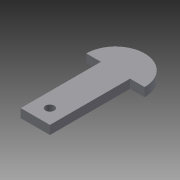
# Autodesk Inventor part: fixing
Saved by Autodesk Inventor 2015 SP2 (Build 190223200, 223)
## iProperties
Created: 2016-03-17
Part Number: fixing
Material: Generic
Document SubType Name: Modeling
Designer: mca20
Density: 1 g/cm^3
Appearance: Default
Author: mca20
Autodesk Inventor part; units mm, degrees
ref_plane "YZ Plane" through (0, 0, 0) normal (1, 0, 0) x (0, 1, 0)
ref_plane "XZ Plane" through (0, 0, 0) normal (0, 1, 0) x (-1, 0, 0)
ref_plane "XY Plane" through (0, 0, 0) normal (0, 0, 1) x (1, 0, 0)
sketch "Sketch1" plane through (0, 0, 0) normal (0, 1, 0) x (-1, 0, 0)
  line L0 (0, 0) -> (10, 0)
  line L1 (10, 0) -> (10, -27.5)
  line L2 (10, -27.5) -> (0, -27.5)
  line L3 (0, -27.5) -> (0, 0)
  line L4 (10, -27.5) -> (15, -27.5)
  line L5 (0, -27.5) -> (-5, -27.5)
  arc A0 (-5, -27.5) -> (15, -27.5) centre (5, -27.5143) ccw
  dimension "d0" = 10
  dimension "d1" = 27.5
  dimension "d2" = 5
  dimension "d3" = 5
  constraints: 12 end point, 2 horizontal, 2 parallel, 2 point on circle, 1 centre point, 1 perpendicular, 1 point on line
  measures "d0" distance of L1.end L2.end
  measures "d1" distance of L0.end L1.end
  measures "d2" distance of L1.end L4.end
  measures "d3" distance of L2.end L5.end
extrude "Extrusion1" add sketch "Sketch1" along normal blind 3
sketch "Sketch2" plane through (0, 3, 0) normal (0, 1, 0) x (1, 0, 0)
  circle A0 centre (-5, 5) radius 1.5
  line L0 (-10, 0) -> (0, 0) projected
  line L1 (-10, 27.5) -> (-10, 0) projected
  dimension "d6" = 3
  dimension "d7" = 5
  dimension "d8" = 5
  constraints: 1 centre point
  measures "d6" diameter of A0
  measures "d7" distance from line of L0 A0.centre
  measures "d8" distance from line of L1 A0.centre
hole "Hole1" at (-5, 3, -5) direction (0, -1, 0) diameter 3 end through all
body "Solid1"
